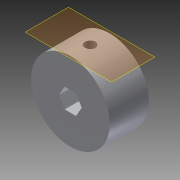
# Autodesk Inventor part: insert
Saved by Autodesk Inventor 2014 SP1 (Build 180222100, 222)
## iProperties
Created: 2014-01-17
Part Number: insert
Material: Aluminum 6061
Document SubType Name: Modeling
Designer: Arpan
Density: 2.71 g/cm^3
Appearance: Aluminum - Flat
Author: Arpan
Autodesk Inventor part; units mm, degrees
ref_plane "YZ Plane" through (0, 0, 0) normal (1, 0, 0) x (0, 1, 0)
ref_plane "XY Plane" through (0, 0, 0) normal (0, 0, 1) x (1, 0, 0)
sketch "Sketch1" plane through (0, 0, 0) normal (0, 0, 1) x (1, 0, 0)
  circle A0 centre (0, 0) radius 25.4
  dimension "d0" = 50.8
  constraints: 1 centre point, 1 coincident
  measures "d0" diameter of A0
extrude "Extrusion1" add sketch "Sketch1" along normal blind 25.4
ref_plane "Work Plane1" through (0, 25.4, 0) normal (0, 1, 0) x (-1, 0, 0)
sketch "Sketch2" plane through (0, 25.4, 0) normal (0, 1, 0) x (-1, 0, 0)
  line L0 (0, 0) -> (0, 12.7)
  circle A0 centre (0, 12.7) radius 3.3782
  dimension "d3" = 12.7
  dimension "d4" = 6.7564
  constraints: 2 end point, 1 centre point, 1 coincident, 1 vertical
  measures "d3" distance of L0.start L0.end
  measures "d4" diameter of A0
extrude "Extrusion2" cut sketch "Sketch2" against normal blind 50.8
sketch "Sketch3" plane through (0, 0, 25.4) normal (0, 0, 1) x (1, 0, 0)
  circle A0 centre (0, 0) radius 25.4 projected
  circle A1 centre (0, 0) radius 6.35
  line L0 (3.6662, 6.35) -> (7.3323, 0)
  line L1 (7.3323, 0) -> (3.6662, -6.35)
  line L2 (3.6662, -6.35) -> (-3.6662, -6.35)
  line L3 (-3.6662, -6.35) -> (-7.3323, 0)
  line L4 (-7.3323, 0) -> (-3.6662, 6.35)
  line L5 (-3.6662, 6.35) -> (3.6662, 6.35)
  point P0 (0, 6.35)
  dimension "d7" = 12.7
  constraints: 12 end point, 2 coincident, 1 midpoint, 1 vertical alignment, 15 other
extrude "Extrusion3" cut sketch "Sketch3" against normal blind 50.8 contours A1 | A1 L0 L1 | A1 L5 L0 | L1 L2 A1 | A1 L4 L5 | L2 L3 A1 | A1 L3 L4
body "Solid1"
